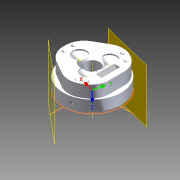
# Autodesk Inventor part: Platfrom_Base_20mm_Rev
Saved by Autodesk Inventor 2011 SP2 (Build 150309200, 309)
## iProperties
Created: 2011-03-08
Part Number: Platfrom_Base_20mm_Rev
Document SubType Name: Modeling
Designer: sungwook
Density: 1.38123 g/cm^3
Material: PET
Mass: 12.1876 g
Surface Area: 32.9133 cm^2
Volume: 8.82374 cm^3
Author: sungwook
Autodesk Inventor part; units mm, degrees
ref_plane "YZ Plane" through (0, 0, 0) normal (1, 0, 0) x (0, 1, 0)
ref_plane "XZ Plane" through (0, 0, 0) normal (0, 1, 0) x (-1, 0, 0)
ref_plane "XY Plane" through (0, 0, 0) normal (0, 0, 1) x (1, 0, 0)
sketch "Sketch1" plane through (0, 0, 0) normal (0, 0, 1) x (1, 0, 0)
  circle A0 centre (0, 0) radius 11.5
  dimension "d0" = 23
  constraints: 1 centre point, 1 coincident
  measures "d0" diameter of A0
extrude "Extrusion1" add sketch "Sketch1" along normal blind 10
sketch "Sketch2" plane through (0, 0, 10) normal (0, 0, 1) x (1, 0, 0)
  circle A0 centre (0, 0) radius 11.5 projected
  circle A1 centre (0, 0) radius 10
  line L0 (0, 0) -> (7.6257, 8.6081)
  line L1 (0, 0) -> (3.642, 10.9081)
  line L2 (-16.73, 0) -> (16.73, 0) projected
  circle A2 centre (3.1669, 9.4853) radius 0.5
  circle A3 centre (6.631, 7.4853) radius 0.5
  line L3 (0, 0) -> (-11.2677, 2.3)
  line L4 (0, 0) -> (-11.2677, -2.3)
  circle A4 centre (-9.798, -2) radius 0.5
  circle A5 centre (-9.798, 2) radius 0.5
  line L5 (0, 0) -> (3.642, -10.9081)
  line L6 (0, 0) -> (7.6257, -8.6081)
  circle A6 centre (6.631, -7.4853) radius 0.5
  circle A7 centre (3.1669, -9.4853) radius 0.5
  dimension "d3" = 20
  dimension "d4" = 48.463
  dimension "d5" = 23.074
  dimension "d6" = 1
  dimension "d7" = 1
  dimension "d178" = 360
  constraints: 12 end point, 7 centre point, 6 point on line, 4 point on circle, 1 coincident, 28 other
  measures "d3" diameter of A1
  measures "d4" angle of L2 L0
  measures "d5" angle of L0 L1
  measures "d6" diameter of A2
  measures "d7" diameter of A3
sketch "Sketch16" plane through (0, 0, 10) normal (0, 0, 1) x (1, 0, 0)
  circle A0 centre (0, 0) radius 11.5 projected
  line L0 (10, 5.6789) -> (10, -5.6789)
  arc A1 (10, -5.6789) -> (10, 5.6789) centre (0, 0) ccw
  dimension "d75" = 10
  constraints: 2 end point, 2 point on circle, 1 centre point, 1 coincident, 1 vertical, 2 other
  measures "d75" distance from line of L0 point (0, 0)
extrude "Extrusion5" cut sketch "Sketch16" against normal through all contours A0 L0 picked at (10.275, -1.294)
pattern_circular "Circular Pattern5" count 3 over 360 about axis through (0, 0, -10) along (0, 0, 1) of "Extrusion5"
fillet "Fillet1" radius 7.62 6 edges at (-9.9181, -5.8208, 5) (-0.0819, -11.4997, 5) (10, -5.6789, 5) (10, 5.6789, 5) (-0.0819, 11.4997, 5) (-9.9181, 5.8208, 5)
sketch "Sketch18" plane through (0, 0, 0) normal (0, 0, -1) x (-1, 0, 0)
  arc A0 (-10, -5.6789) -> (0.0819, -11.4997) centre (0, 0) ccw projected
  circle A1 centre (0, 0) radius 7
  line L0 (16.73, 0) -> (-16.73, 0) projected
  point P0 (-7, 0)
  point P1 (7, 0)
  dimension "d112" = 14
  constraints: 1 coincident, 1 horizontal alignment, 2 other
hole "Attachment Hole M2.5" at (-7, 0, 0) direction (0, 0, 1) diameter 1.7018 depth 4
pattern_circular "Circular Pattern7" count 3 over 360 about axis through (0, 0, -10) along (0, 0, 1) of "Attachment Hole M2.5"
pattern_circular "Circular Pattern8" count 3 over 360 about axis through (0, 0, -10) along (0, 0, 1) of "Attachment Hole M2.5"
ref_plane "Work Plane7" through (6.631, 7.4853, 10) normal (0.7485281, -0.663103, 0) x (-0.663103, -0.7485281, 0)
ref_plane "Work Plane8" through (3.1669, 9.4853, 10) normal (0.9485281, -0.3166929, 0) x (-0.3166929, -0.9485281, 0)
sketch "Sketch21" plane through (6.631, 7.4853, 10) normal (0.7485281, -0.663103, 0) x (-0.663103, -0.7485281, 0)
  line L0 (10, 0) -> (-1.5, 0) projected
  line L1 (0, 0) -> (-1.5543, 7.7083)
  point P0 (10, 10)
  dimension "d147" = 101.4
  constraints: 2 end point, 1 point on line
  measures "d147" angle of L1 L0
hole "Hole12" at (6.631, 7.4853, 10) direction (0.1310672, 0.1479521, -0.9802712) diameter 0.5 end through all countersink diameter 1.5 countersink angle 90
sketch "Sketch22" plane through (6.631, 7.4853, 10) normal (0.7485281, -0.663103, 0) x (-0.663103, -0.7485281, 0)
  line L0 (0, 0) -> (0, 0) projected
  line L1 (0, 0) -> (0, 0) projected
  line L2 (0.1462, 0.5395) -> (-0.3439, 0.4407) projected
  line L3 (0, 0) -> (0.7352, 0.1482) projected
  line L4 (0.7352, 0.1482) -> (0.1462, 0.5395) projected
  line L5 (21.0937, 0) -> (-1.0937, 0) projected
  line L6 (0.7352, 0.1482) -> (2.8954, -1.287)
  line L7 (2.8954, -1.287) -> (0, 0)
  line L8 (2.0001, -9.9194) -> (-2.9069, 14.4168) projected
  point P0 (10, 10)
  constraints: 4 end point, 1 collinear
revolve "Revolution5" cut sketch "Sketch22" angle 360 about axis through (6.631, 7.4853, 10) along (0.1310672, 0.1479521, -0.9802712) contours L6 L5 L3 | L5 L6 L7
sketch "Sketch23" plane through (3.1669, 9.4853, 10) normal (0.9485281, -0.3166929, 0) x (-0.3166929, -0.9485281, 0)
  line L0 (0, 0) -> (-1.0061, 4.9898)
  line L1 (10, 0) -> (-1.5, 0) projected
  point P0 (10, 10)
  dimension "d158" = 101.4
  constraints: 2 end point, 1 point on line
  measures "d158" angle of L0 L1
hole "Hole13" at (3.1669, 9.4853, 10) direction (0.0625967, 0.1874835, -0.9802712) diameter 0.5 end through all countersink diameter 1.5 countersink angle 90
sketch "Sketch24" plane through (3.1669, 9.4853, 10) normal (0.9485281, -0.3166929, 0) x (-0.3166929, -0.9485281, 0)
  line L0 (0.1462, 0.5395) -> (0.7352, 0.1482) projected
  line L1 (0.7352, 0.1482) -> (0, 0) projected
  line L2 (10, 0) -> (-0.58, 0) projected
  line L3 (0.7352, 0.1482) -> (2.2664, -0.8691)
  line L4 (2.2664, -0.8691) -> (0, 0)
  line L5 (-2.7951, 13.8619) -> (1.8072, -8.9629) projected
  point P0 (10, 10)
  constraints: 4 end point, 1 collinear
revolve "Revolution6" cut sketch "Sketch24" angle 360 about axis through (3.4856, 10.4396, 5.0102) along (-0.0625967, -0.1874835, 0.9802712)
pattern_circular "Circular Pattern Top Hole" count 3 over 360 about axis through (0, 0, -10) along (0, 0, 1) of "Hole13", "Revolution6", "Hole12", "Revolution5"
sketch "Sketch25" plane through (0, 0, 0) normal (0, 0, -1) x (-1, 0, 0)
  line L0 (-10, 5.6789) -> (-10, -5.6789) projected
  line L1 (-12.3287, 5) -> (-9.5, 5)
  line L2 (-9.5, 5) -> (-9.5, -5)
  line L3 (-9.5, -5) -> (-12.3287, -5)
  line L4 (-12.3287, -5) -> (-12.3287, 5)
  point P0 (-10, 3.0643)
  point P1 (-10, -3.0643)
  point P2 (-12.3287, 0)
  dimension "d172" = 10
  dimension "d173" = 0.5
  constraints: 8 end point, 2 parallel, 1 horizontal, 1 midpoint, 1 perpendicular
  measures "d172" distance of L3.end L1.start
  measures "d173" distance between parallel lines of L2 L0
extrude "Extrusion Side" [suppressed]
hole "Center Hole" at (0, 0, 10) direction (0, 0, -1) diameter 6 end through all
hole "Center Bottom Bore" at (0, 0, 0) direction (0, 0, 1) diameter 11 depth 2
sketch "Sketch35" plane through (0, 0, 0) normal (0, 0, -1) x (-1, 0, 0)
  line L0 (16.73, 0) -> (-16.73, 0) projected
  circle A0 centre (-6.1536, 1.5672) radius 1.4986
  circle A1 centre (0, 0) radius 5.5 projected
  arc A2 (-4.3385, 10.6502) -> (-7.0541, 9.0824) centre (0, 0) ccw projected
  line L1 (2.921, 5.0593) -> (0, 0)
  dimension "d246" = 2.9972
  dimension "d255" = 6.35
  dimension "d324" = 60
  dimension "d325" = 5.842
  constraints: 2 end point, 1 centre point
  measures "d246" diameter of A0
  measures "d255" distance of A0.centre A1.centre
  measures "d324" angle of L0 L1
  measures "d325" distance of L1.start A1.centre
hole "Jig Hole" at (-2.921, 5.0593, 0) direction (0, 0, 1) diameter 2.9972 depth 5
sketch "Sketch37" plane through (0, 0, 0) normal (0, 0, -1) x (-1, 0, 0)
  circle A0 centre (0, 0) radius 9.64
  line L0 (16.73, 0) -> (-16.73, 0) projected
  point P0 (9.64, 0)
  dimension "d277" = 19.28
  dimension "d288" = 9.64
  constraints: 1 centre point
  measures "d277" diameter of A0
  measures "d288" distance of A0.centre point (9.64, 0)
hole "PCB Attachment" at (-9.64, 0, 0) direction (0, 0, 1) diameter 1.1938 depth 7.112
pattern_circular "Circular Pattern11" count 3 over 360 about axis through (0, 0, -10) along (0, 0, 1) of "PCB Attachment"
sketch "Sketch39" plane through (0, 0, 10) normal (0, 0, 1) x (1, 0, 0)
  arc A0 (4.3385, -10.6502) -> (7.0541, -9.0824) centre (0, 0) ccw projected
  circle A1 centre (0, 0) radius 5.2324
  point P0 (-5.2324, -0.0001)
  dimension "d290" = 10.4648
  constraints: 1 coincident, 3 other
hole "Spring Guide Hole" at (-5.2324, -0.0001, 10) direction (0, 0, -1) diameter 5.588 depth 0.508 tip angle 118
hole "Spring Hole" at (-5.2324, -0.0001, 10) direction (0, 0, -1) diameter 0.5 end through all
pattern_circular "Spring r Pattern12" count 3 over 360 about axis through (0, 0, -10) along (0, 0, 1) of "Spring Guide Hole", "Spring Hole"
chamfer "Chamfer Center" distance 1.524 angle 45 4 edges at (-1.6233, -2.5229, 10) (0.1444, -2.9965, 10) (-1.5, 2.5981, 10) (3, 0, 10)
sketch "Sketch43" plane through (0, 0, 10) normal (0, 0, 1) x (1, 0, 0)
  arc A0 (4.0038, -2.1062) -> (4.0037, 2.1063) centre (0, 0) ccw projected
  arc A1 (-3.826, -2.4143) -> (-0.1777, -4.5205) centre (0, 0) ccw projected
  line L0 (6.35, 3.81) -> (7.62, 3.81)
  line L1 (7.62, 3.81) -> (7.62, -3.81)
  line L2 (7.62, -3.81) -> (6.35, -3.81)
  line L3 (6.35, -3.81) -> (6.35, 3.81)
  point P0 (6.35, 0)
  dimension "d316" = 7.62
  dimension "d317" = 1.27
  dimension "d318" = 6.35
  constraints: 8 end point, 2 parallel, 1 horizontal, 1 horizontal alignment, 1 midpoint, 1 perpendicular
  measures "d316" distance of L1.end L0.end
  measures "d317" distance of L0.end L0.start
  measures "d318" distance from line of L3 A0.centre
extrude "PCB Slot" cut sketch "Sketch43" against normal through all
chamfer "Chamfer3" distance 1.27 angle 45 1 edges at (6.35, 0, 10)
sketch "Sketch47" plane through (0, 0, 0) normal (0, 0, -1) x (-1, 0, 0)
  arc A0 (11.3926, 1.5679) -> (7.6538, 7.1281) centre (3.8438, 0.529) ccw projected
  line L0 (7.6538, 7.1281) -> (2.3462, 10.1924) projected
  arc A1 (2.3462, 10.1924) -> (-4.3385, 10.6502) centre (-1.4638, 3.5933) ccw projected
  arc A2 (-4.3385, 10.6502) -> (-7.0541, 9.0824) centre (0, 0) ccw projected
  arc A3 (-7.0541, 9.0824) -> (-10, 3.0643) centre (-2.38, 3.0643) ccw projected
  line L1 (-10, 3.0643) -> (-10, -3.0643) projected
  arc A4 (-10, -3.0643) -> (-7.0541, -9.0824) centre (-2.38, -3.0643) ccw projected
  arc A5 (-7.0541, -9.0824) -> (-4.3385, -10.6502) centre (0, 0) ccw projected
  arc A6 (-4.3385, -10.6502) -> (2.3462, -10.1924) centre (-1.4638, -3.5933) ccw projected
  line L2 (2.3462, -10.1924) -> (7.6538, -7.1281) projected
  arc A7 (7.6538, -7.1281) -> (11.3926, -1.5679) centre (3.8438, -0.529) ccw projected
  arc A8 (11.3926, -1.5679) -> (11.3926, 1.5679) centre (0, 0) ccw projected
  arc A9 (1.4431, 5.3073) -> (3.8747, 3.9034) centre (0, 0) ccw projected
  circle A10 centre (0, 0) radius 11.95
  dimension "d338" = 23.9
  constraints: 1 centre point, 1 coincident
  measures "d338" diameter of A10
extrude "Extrusion11" add sketch "Sketch47" against normal blind 5
sketch "Sketch48" plane through (0, 0, 0) normal (0, 0, -1) x (-1, 0, 0)
  line L0 (-7.62, 3.81) -> (-6.35, 3.81) projected
  arc A0 (1.4431, 5.3073) -> (3.8747, 3.9034) centre (0, 0) ccw projected
  circle A1 centre (-9.62, 0) radius 0.889
  circle A2 centre (-6.85, 5.5) radius 0.889
  circle A3 centre (-6.85, -5.5) radius 0.889
  line L1 (-7.62, 3.81) -> (-6.35, 3.81)
  line L2 (-6.35, 3.81) -> (-6.35, -3.81)
  line L3 (-6.35, -3.81) -> (-7.62, -3.81)
  line L4 (-7.62, -3.81) -> (-7.62, 3.81)
  line L5 (0, 0) -> (-9.6022, 11.4435)
  line L6 (0, 0) -> (-9.6022, -11.4435)
  arc A4 (-9.6022, 11.4435) -> (-9.6022, -11.4435) centre (0, 0) ccw
  line L7 (17.3277, 0) -> (-20.3161, 0) projected
  dimension "d350" = 100
  dimension "d352" = 2
  constraints: 12 end point, 4 centre point, 2 point on circle, 1 coincident, 1 point on line, 1 other
  measures "d350" angle of L6 L5
  measures "d352" distance from line of L4 A1.centre
extrude "Extrusion12" cut sketch "Sketch48" against normal blind 0.6 contours L4 L7 A1 A4 L5 A0 L2 L0 | L4 L3 L2 L7 A0 L6 A4 A1 | L7 A1 | A1 L7 | L7 L6 A0 | A0 L5 L7 | A2 | A3 picked at (-3.6232, -0.3968)
hole "Hole27" at (6.85, 5.5, 0) at (9.62, 0, 0) at (6.85, -5.5, 0) direction (0, 0, 1) diameter 1.1938 depth 3
sketch "Sketch50" plane through (0, 0, 0) normal (0, 0, -1) x (-1, 0, 0)
  circle A0 centre (-3.5, 6.0622) radius 0.8509 projected
  circle A1 centre (-3.5, -6.0622) radius 0.8509 projected
  circle A2 centre (7, 0) radius 0.8509 projected
  circle A3 centre (9.64, 0) radius 0.5969 projected
  circle A4 centre (-4.82, -8.3485) radius 0.5969 projected
  circle A5 centre (-4.82, 8.3485) radius 0.5969 projected
  line L0 (-3.5353, -4.2132) -> (-7.6813, -9.1542) projected
  arc A6 (-7.6813, -9.1542) -> (-7.6813, 9.1542) centre (0, 0) ccw projected
  line L1 (-7.6813, 9.1542) -> (-3.5353, 4.2132) projected
  arc A7 (1.4431, 5.3073) -> (-3.5353, 4.2132) centre (0, 0) ccw projected
  arc A8 (3.8747, 3.9034) -> (1.4431, 5.3073) centre (2.921, 5.0593) ccw projected
  arc A9 (-3.5353, -4.2132) -> (3.8747, 3.9034) centre (0, 0) ccw projected
  arc A10 (-7.6813, 9.1542) -> (-7.6813, -9.1542) centre (0, 0) ccw projected
  line L2 (16.73, 0) -> (-16.73, 0) projected
  line L3 (0, -16.73) -> (0, 16.73) projected
  point P0 (0, 11.95)
  constraints: 1 coincident, 1 point on circle, 1 point on line
sketch "Sketch51" plane through (0, 0, 0) normal (0, 0, -1) x (-1, 0, 0)
  circle A0 centre (-3.5, 6.0622) radius 0.8509 projected
  circle A1 centre (-3.5, -6.0622) radius 0.8509 projected
  circle A2 centre (7, 0) radius 0.8509 projected
  circle A3 centre (9.64, 0) radius 0.5969 projected
  circle A4 centre (-4.82, -8.3485) radius 0.5969 projected
  circle A5 centre (-4.82, 8.3485) radius 0.5969 projected
  line L0 (-3.5353, -4.2132) -> (-7.6813, -9.1542) projected
  arc A6 (-7.6813, -9.1542) -> (-7.6813, 9.1542) centre (0, 0) ccw projected
  line L1 (-7.6813, 9.1542) -> (-3.5353, 4.2132) projected
  arc A7 (1.4431, 5.3073) -> (-3.5353, 4.2132) centre (0, 0) ccw projected
  arc A8 (3.8747, 3.9034) -> (1.4431, 5.3073) centre (2.921, 5.0593) ccw projected
  arc A9 (-3.5353, -4.2132) -> (3.8747, 3.9034) centre (0, 0) ccw projected
  line L2 (-15.1503, 18.0555) -> (15.1503, -18.0555) projected
  point P0 (7.6813, -9.1542)
  constraints: 1 point on circle, 1 point on line
ref_plane "Work Plane11" through (-7.6813, -9.1542, 0) normal (-0.6427876, -0.7660444, 0) x (0.7660444, -0.6427876, 0)
sketch "Sketch52" plane through (-7.6813, -9.1542, 0) normal (-0.6427876, -0.7660444, 0) x (0.7660444, -0.6427876, 0)
  line L0 (0, -2.0004) -> (0, 12.0025) projected
  line L1 (-28.6889, 0) -> (28.0867, 0) projected
  line L2 (-11.95, 5) -> (11.95, 5) projected
  point P0 (0, 0)
  point P1 (0, 2.5)
  dimension "d365" = 5
  dimension "d366" = 2.5
  constraints: 1 point on line
  measures "d365" distance between parallel lines of L1 L2
  measures "d366" distance from line of L1 point (0, 2.5)
hole "Hole28" at (-7.6813, -9.1542, 2.5) direction (0.6427876, 0.7660444, 0) diameter 1.1938 depth 3
mirror "Mirror2" about plane through (0, 0, 0) normal (0, 1, 0) of "Hole28"
ref_plane "Work Plane13" through (2.891, 11.595, 0) normal (0.2419219, 0.9702957, 0) x (-0.9702957, 0.2419219, 0)
sketch "Sketch53" plane through (2.891, 11.595, 0) normal (0.2419219, 0.9702957, 0) x (-0.9702957, 0.2419219, 0)
  line L0 (-11.95, 5) -> (11.95, 5) projected
  line L1 (-5.2385, 0.6) -> (-11.95, 0.6) projected
  line L2 (0, 12.0025) -> (0, -2.0004) projected
  line L3 (11.95, 0) -> (-9.6678, 0) projected
  point P0 (0, 0)
  point P1 (-9.6678, 0.6)
  point P2 (0, 2.5)
  point P3 (-5.2385, 0)
  dimension "d380" = 2.5
  constraints: 1 point on line
  measures "d380" distance from line of L3 point (0, 2.5)
hole "Hole29" at (2.891, 11.595, 2.5) direction (-0.2419219, -0.9702957, 0) diameter 1.1938 depth 3
mirror "Mirror3" about plane through (0, 0, 0) normal (0, 1, 0) of "Hole29"
sketch "Sketch54" plane through (-7.6538, 7.1281, 10) normal (-0.5, 0.8660254, 0) x (0.8660254, 0.5, 0)
  line L0 (3.0643, 12.0004) -> (3.0643, -2.0025) projected
  point P0 (0, 0)
  point P1 (3.0643, 10)
  point P2 (3.0643, 2.5)
  dimension "d388" = 2.5
  constraints: 1 point on line
  measures "d388" vertical distance of point (3.064, 2.5) point (0, 0)
hole "Hole30" at (-5, 8.6603, 7.5) direction (0.5, -0.8660254, 0) diameter 1.1938 depth 3
mirror "Mirror4" about plane through (0, 0, 0) normal (0, 1, 0) of "Hole30"
ref_plane "Work Plane12" through (0, 0, 0) normal (0, 1, 0) x (-1, 0, 0)
equation "\"d0\" = baseOD"
equation "\"d3\" = baseD"
equation "\"d4\" = baseTh0"
equation "\"d5\" = baseTh1"
equation "\"baseD\" = 20"
equation "\"springBaseD\" = 8"
equation "\"baseOD\" = 23"
equation "\"CSpringOD\" = 5.537"
equation "\"lFlexure\" = 6.7"
equation "\"springUnderCut\" = 9.2"
equation "\"GuideRod\" = 2"
equation "\"dMotor\" = 1.44"
equation "\"dM2Y\" = 7.00349"
equation "\"GuideTubingOD\" = 4"
equation "\"springInitL\" = 12.7"
equation "\"springL\" = 30.86629"
equation "\"dM1Xt\" = 6.59227"
equation "\"dM2Yt\" = 5.49055"
equation "\"lFlexureOffset\" = 3.7"
equation "\"springDeform\" = 18.16629"
equation "\"dM1Y\" = 2.34012"
equation "\"dM2Xt\" = -3.67462"
equation "\"topH\" = 21.66629"
equation "\"springLO\" = 33.86629"
equation "\"GuideTubingID\" = 2"
equation "\"dM1X\" = 6.73587"
equation "\"lMotor\" = 22.35"
equation "\"CSpringCD\" = 0.254"
equation "\"dM2X\" = -1.34133"
equation "\"dM1Yt\" = -0.43704"
equation "\"CSpringID\" = 5.029"
equation "\"springTopD\" = 8"
equation "\"springLset\" = 3.5"
equation "\"baseInitD\" = 4"
equation "\"topD\" = 14"
equation "\"topInitD\" = 4"
equation "\"dFlexure\" = 0.38"
equation "\"topTh0\" = 16.60155deg"
equation "\"topTh1\" = 86.796901deg"
equation "\"baseTh0\" = 48.463deg"
equation "\"baseTh1\" = 23.0739deg"
body "Solid1"
